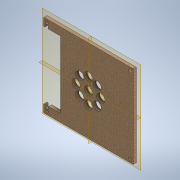
# Autodesk Inventor part: MDF_Top_Big_Mic
Saved by Autodesk Inventor 2021 (Build 250183000, 183)
## iProperties
Created: 2021-02-17
Part Number: MDF_Top_Big_Mic
Material: MDF Medium Density Fiberboard
Document SubType Name: Modeling
Designer: negt20
Density: 0.8 g/cm^3
Appearance: Cardboard - Corrugated
Author: negt20
Autodesk Inventor part; units mm, degrees
sketch "Sketch1" plane through (0, 0, 0) normal (0, 0, 1) x (1, 0, 0)
  line L0 (-91.5, 84.5) -> (91.5, 84.5)
  line L1 (91.5, 84.5) -> (91.5, -84.5)
  line L2 (91.5, -84.5) -> (-91.5, -84.5)
  line L3 (-91.5, -84.5) -> (-91.5, 84.5)
  point P0 (0, 84.5)
  point P1 (0, 0)
  point P2 (-91.5, 0)
  dimension "d0" = 183
  dimension "d1" = 169
  constraints: 8 end point, 2 midpoint, 2 parallel, 1 horizontal, 1 horizontal alignment, 1 perpendicular, 1 vertical alignment
  measures "d0" distance of L1.end L2.end
  measures "d1" distance of L0.end L1.end
extrude "Extrusion1" add sketch "Sketch1" along normal blind 6
sketch "Sketch2" plane through (0, 0, 6) normal (0, 0, 1) x (1, 0, 0)
  line L0 (-91.5, -84.5) -> (91.5, -84.5) projected
  line L1 (0, -84.5) -> (-85, -84.5) construction
  line L2 (-85, -84.5) -> (-85, -78) construction
  circle A0 centre (-85, -78) radius 3.25
  line L3 (-85, -78) -> (-85, -74) construction
  line L4 (-88.25, -68) -> (-81.75, -68)
  line L5 (-81.75, -68) -> (-81.75, -74)
  line L6 (-81.75, -74) -> (-88.25, -74)
  line L7 (-88.25, -74) -> (-88.25, -68)
  point P0 (0, 0)
  point P1 (40.5, -62.5)
  dimension "d37" = 85
  dimension "d38" = 6.5
  dimension "d39" = 6.5
  dimension "d44" = 4
  dimension "d45" = 6.5
  dimension "d46" = 6
  constraints: 14 end point, 3 coincident, 2 midpoint, 2 parallel, 2 perpendicular, 1 centre point, 1 horizontal, 1 vertical
  measures "d37" distance of L1.start L1.end
  measures "d38" distance of L1.end L2.end
  measures "d39" diameter of A0
  measures "d44" distance of L3.start L3.end
  measures "d45" distance of L5.end L6.end
  measures "d46" distance of L4.end L5.end
extrude "Extrusion2" cut sketch "Sketch2" against normal blind 6 contours A0
mirror "Mirror3" about plane through (0, 0, 0) normal (1, 0, 0) of "Extrusion2"
mirror "Mirror7" about plane through (0, 0, 0) normal (0, 1, 0) of "Extrusion2", "Mirror3"
sketch "Sketch7" plane through (0, 0, 6) normal (0, 0, 1) x (1, 0, 0)
  line L0 (-91.5, 84.5) -> (-91.5, -84.5) projected
  line L1 (-91.5, 68) -> (-57, 68)
  line L2 (-57, 68) -> (-57, -68)
  line L3 (-57, -68) -> (-91.5, -68)
  line L4 (-91.5, -68) -> (-91.5, 68)
  point P0 (0, 0)
  point P1 (-91.5, 0)
  point P2 (-91.5, 0)
  dimension "d40" = 34.5
  dimension "d41" = 136
  constraints: 8 end point, 2 midpoint, 2 parallel, 1 coincident, 1 horizontal, 1 perpendicular, 1 point on line
  measures "d40" distance of L2.end L3.end
  measures "d41" distance of L1.end L2.end
extrude "Extrusion6" cut sketch "Sketch7" against normal blind 10
sketch "Sketch8" plane through (0, 0, 6) normal (0, 0, 1) x (1, 0, 0)
  circle A0 centre (-85, -78) radius 3.25 projected
  line L0 (-85, -78) -> (-85, -73.75) construction
  line L1 (-88.125, -68) -> (-81.875, -68)
  line L2 (-81.875, -68) -> (-81.875, -73.75)
  line L3 (-81.875, -73.75) -> (-88.125, -73.75)
  line L4 (-88.125, -73.75) -> (-88.125, -68)
  point P0 (0, 0)
  dimension "d47" = 4.25
  dimension "d48" = 6.25
  dimension "d49" = 5.75
  constraints: 10 end point, 2 coincident, 2 parallel, 1 horizontal, 1 midpoint, 1 perpendicular, 1 vertical
  measures "d47" distance of L0.start L0.end
  measures "d48" distance of L2.end L3.end
  measures "d49" distance of L1.end L2.end
extrude "Extrusion7" cut sketch "Sketch8" against normal blind 6 contours L1 L2 L3 L4
mirror "Mirror8" about plane through (0, 0, 0) normal (0, 1, 0) of "Extrusion7"
fillet "Fillet5" radius 1 12 edges at (-91.5, -84.5, 3) (91.5, -84.5, 3) (-57, -68, 3) (91.5, 84.5, 3) (-91.5, 84.5, 3) (-91.5, 68, 3) (-57, 68, 3) (-81.875, 68, 3) (-88.125, 68, 3) (-81.875, -68, 3) (-91.5, -68, 3) (-88.125, -68, 3)
sketch "Sketch10" plane through (0, 0, 6) normal (0, 0, 1) x (1, 0, 0)
  line L0 (-57, 44.5) -> (57, 44.5) construction
  line L1 (57, 44.5) -> (57, -44.5) construction
  line L2 (57, -44.5) -> (-57, -44.5) construction
  line L3 (-57, -44.5) -> (-57, 44.5) construction
  line L4 (-57, 67) -> (-57, -67) projected
  line L5 (-57, 44.5) -> (57, -44.5) construction
  circle A0 centre (0, 0) radius 8.25
  line L6 (0, 0) -> (0, 25) construction
  circle A1 centre (0, 25) radius 8.25
  point P0 (-57, 0)
  point P1 (-57, 0)
  point P2 (-57, 0)
  dimension "d53" = 114
  dimension "d54" = 89
  dimension "d55" = 16.5
  dimension "d56" = 25
  dimension "d57" = 16.5
  constraints: 12 end point, 4 coincident, 3 midpoint, 2 centre point, 2 parallel, 1 horizontal, 1 perpendicular, 1 vertical
  measures "d53" distance of L1.end L2.end
  measures "d54" distance of L0.end L1.end
  measures "d55" diameter of A0
  measures "d56" distance of L6.start L6.end
  measures "d57" diameter of A1
extrude "Extrusion8" cut sketch "Sketch10" against normal through all
pattern_circular "Circular Pattern1" count 8 over 360 about axis through (0, 0, 6) along (0, 0, -1) of "Extrusion8"
equation "\"d7\" = d46"
body "Solid1"
